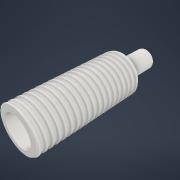
# Autodesk Inventor part: screw
Saved by Autodesk Inventor 2022.1 (Build 261234020, 234B)
## iProperties
Created: 2021-12-02
Part Number: screw
Material: Generic
Document SubType Name: Modeling
Designer: PaulT
Density: 1 g/cm^3
Appearance: Steel
Author: PaulT
Autodesk Inventor part; units mm, degrees
ref_plane "YZ Plane" through (0, 0, 0) normal (1, 0, 0) x (0, 1, 0)
ref_plane "XZ Plane" through (0, 0, 0) normal (0, 1, 0) x (-1, 0, 0)
ref_plane "XY Plane" through (0, 0, 0) normal (0, 0, 1) x (1, 0, 0)
sketch "Sketch1" plane through (0, 0, 0) normal (1, 0, 0) x (0, 1, 0)
  line L0 (0, 3.8) -> (0, -22.8) projected
  line L1 (0, 0) -> (2.9, 0)
  line L2 (2.9, 0) -> (2.9, -14)
  line L3 (2.9, -14) -> (1.4, -15.5)
  line L4 (1.4, -15.5) -> (1.4, -19)
  line L5 (1.4, -19) -> (0, -19)
  line L6 (-0.58, 0) -> (3.48, 0) projected
  point P0 (0.7, -19)
  dimension "d6" = 19
  dimension "d7" = 1.4
  dimension "d8" = 2.9
  dimension "d9" = 1.5
  dimension "d10" = 3.5
  constraints: 10 end point, 2 perpendicular, 2 point on line, 1 collinear, 1 horizontal, 1 midpoint, 1 parallel
  measures "d6" distance from line of L1 point (0.7, -19)
  measures "d7" distance of L4.end L5.end
  measures "d8" distance between parallel lines of L0 L2
  measures "d9" horizontal distance of L2.end L3.end
  measures "d10" distance of L3.end L4.end
revolve "Revolution1" add sketch "Sketch1" angle 360 about axis through (0, 0, 0) along (0, 0, -1)
sketch "Sketch2" plane through (0, 0, 0) normal (0, 0, 1) x (1, 0, 0)
  circle A0 centre (0, 0) radius 1.4 projected
  circle A1 centre (0, 0) radius 2
  dimension "d12" = 4
  constraints: 1 centre point, 1 coincident
  measures "d12" diameter of A1
extrude "Extrusion1" cut sketch "Sketch2" against normal blind 13 contours A0 | A1
sketch "Sketch3" plane through (0, 0, -19) normal (0, 0, -1) x (-1, 0, 0)
  circle A0 centre (0, 0) radius 1
  dimension "d15" = 2
  constraints: 1 centre point, 1 coincident
  measures "d15" diameter of A0
extrude "Extrusion2" cut sketch "Sketch3" against normal through all
sketch "Sketch4" plane through (0, 0, 0) normal (1, 0, 0) x (0, 1, 0)
  circle A0 centre (3, 1) radius 0.25
  line L0 (-2.9, 0) -> (2.9, 0) projected
  line L1 (0, 6.9267) -> (0, -22.0855) construction
  point P0 (0, 0)
  dimension "d18" = 0.5
  dimension "d19" = 1
  dimension "d20" = 3
  constraints: 2 end point, 1 centre point, 1 vertical
  measures "d18" diameter of A0
  measures "d19" distance from line of L0 A0.centre
  measures "d20" horizontal distance of A0.centre point (0, 0)
coil "Coil1" sketch "Sketch4" operation cut axis through (0, 0, 6.9267) along (0, 0, -1) pitch 0.75 turns 22 hand right
fillet "Fillet1" radius 0.1 10 edges at (2.3753, 1.6637, -13.8854) (-1.6637, -2.3753, -13.9271) (-2.6285, 1.2251, -0.1354) (2.8889, -0.2532, -0.1771) (0, -1.4, -19) (-2.6285, 1.2252, 0) (0.2532, 2.8889, 0) (-1.2141, -2.5502, 0) (2.7495, -0.1894, 0) (0, -1.4, -15.5)
body "Solid1"
